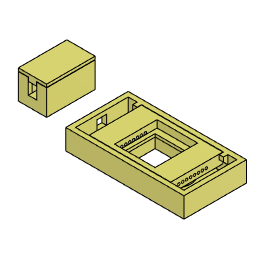
ESP07 Breadboard Adapter (Autodesk Fusion 360 design; units mm, degrees)
Autodesk Fusion 360 part; units mm, degrees
sketch "Footprint" plane through (0, 0, 0) normal (0, 0, 1) x (1, 0, 0)
  line L0 (21, 13.4625) -> (-21, 13.4625)
  line L1 (-21, 13.4625) -> (-21, -13.4625)
  line L2 (-21, -13.4625) -> (21, -13.4625)
  line L3 (21, -13.4625) -> (21, 13.4625)
  line L4 (21, 13.4625) -> (-21, -13.4625) construction
  line L5 (-21, 13.4625) -> (21, -13.4625) construction
  line L6 (10.45, 10.9625) -> (-10.45, 10.9625)
  line L7 (-10.45, 10.9625) -> (-10.45, -10.9625)
  line L8 (-10.45, -10.9625) -> (10.45, -10.9625)
  line L9 (10.45, -10.9625) -> (10.45, 10.9625)
  line L10 (10.45, 10.9625) -> (-10.45, -10.9625) construction
  line L11 (-10.45, 10.9625) -> (10.45, -10.9625) construction
  line L12 (-8.45, 7.9625) -> (8.45, 7.9625)
  line L13 (8.45, 7.9625) -> (8.45, -7.9625)
  line L14 (8.45, -7.9625) -> (-8.45, -7.9625)
  line L15 (-8.45, -7.9625) -> (-8.45, 7.9625)
  line L16 (-8.45, 7.9625) -> (8.45, -7.9625) construction
  line L17 (8.45, 7.9625) -> (-8.45, -7.9625) construction
  dimension "d16" = 21.925
  dimension "d17" = 20.9
  dimension "d18" = 2.5
  dimension "d19" = 10.55
  dimension "d20" = 3
  dimension "d21" = 2
  constraint perpendicular L0 L1
  constraint parallel L0 L2
  constraint parallel L1 L3
  constraint horizontal L0
  constraint coincident L4 origin
  constraint coincident L5 origin
  constraint perpendicular L6 L7
  constraint parallel L6 L8
  constraint parallel L7 L9
  constraint horizontal L6
  constraint coincident L10 origin
  constraint coincident L11 origin
  constraint perpendicular L12 L13
  constraint parallel L12 L14
  constraint parallel L13 L15
  constraint horizontal L12
  constraint coincident L16 origin
  constraint coincident L17 origin
  measures "d16" distance of L6.start L8.end
  measures "d17" distance of L7.end L8.end
  measures "d18" distance of L0 L6
  measures "d19" distance of L3 L9
  measures "d20" distance of L6 L12
  measures "d21" distance of L9 L13
extrude "Extrude1" add sketch "Footprint" against normal blind 1.5 contours L0 L1 L2 L3 | L6 L7 L8 L9 makes body 1
extrude "Extrude2" add sketch "Footprint" along normal blind 3.76 contours L0 L1 L2 L3 bodies 1
sketch "PogoPin Holes Profile" plane through (-10.45, 0, 0) normal (1, 0, 0) x (0, 1, 0)
  line L0 (-10.9625, 0) -> (10.9625, 0) construction
  line L1 (10.9625, 0) -> (10.9625, 3.76) construction
  line L2 (10.9625, 3.76) -> (-10.9625, 3.76) construction
  line L3 (-10.9625, 3.76) -> (-10.9625, 0) construction
  circle A0 centre (-9.2555, 0.8) radius 0.655
  circle A1 centre (-7.2355, 0.8) radius 0.655
  circle A2 centre (-5.2155, 0.8) radius 0.655
  circle A3 centre (-3.1955, 0.8) radius 0.655
  circle A4 centre (-1.1755, 0.8) radius 0.655
  circle A5 centre (0.8445, 0.8) radius 0.655
  circle A6 centre (2.8645, 0.8) radius 0.655
  circle A7 centre (4.8845, 0.8) radius 0.655
  dimension "d26" = 1.707
  dimension "d27" = 0.8
  dimension "d28" = 1.31
  dimension "d31" = 2.02
  dimension "d32" = 0
  measures "d26" distance of L3 A0.centre
  measures "d27" distance of L0 A0.centre
  measures "d28" diameter of A0
extrude "Extrude3" cut sketch "PogoPin Holes Profile" along normal through all and the other way through all bodies 1
sketch "Protector Sleve Profile" plane through (0, 0, -1.5) normal (0, 0, -1) x (1, 0, 0)
  line L0 (-28, 13.6175) -> (28, 13.6175)
  line L1 (28, 13.6175) -> (28, -13.6175)
  line L2 (28, -13.6175) -> (-28, -13.6175)
  line L3 (-28, -13.6175) -> (-28, 13.6175)
  line L4 (-28, 13.6175) -> (28, -13.6175) construction
  line L5 (28, 13.6175) -> (-28, -13.6175) construction
  line L6 (21, 13.4625) -> (-21, 13.4625)
  line L7 (30.5, -16.1175) -> (-30.5, -16.1175)
  line L8 (-30.5, -16.1175) -> (-30.5, 16.1175)
  line L9 (-30.5, 16.1175) -> (30.5, 16.1175)
  line L10 (30.5, 16.1175) -> (30.5, -16.1175)
  line L11 (21, -13.4625) -> (21, 13.4625)
  line L12 (-8.45, -7.9625) -> (-8.45, 7.9625)
  line L13 (8.45, 7.9625) -> (8.45, -7.9625)
  line L14 (8.45, -7.9625) -> (-8.45, -7.9625)
  line L15 (-8.45, 7.9625) -> (8.45, 7.9625)
  line L16 (-11.45, -9.1625) -> (11.45, -9.1625)
  line L17 (-11.45, 9.1625) -> (11.45, 9.1625)
  line L18 (0, -9.1625) -> (0, 9.1625) construction
  arc A0 (-11.45, 9.1625) -> (-11.45, -9.1625) centre (-7.9401, 0) ccw
  arc A1 (11.45, -9.1625) -> (11.45, 9.1625) centre (7.9401, 0) ccw
  point P0 (-21, 13.4625)
  point P1 (21, 13.4625)
  point P2 (21, -13.4625)
  point P3 (-21, -13.4625)
  point P4 (8.45, 7.9625)
  point P5 (-8.45, 7.9625)
  point P6 (-8.45, -7.9625)
  point P7 (8.45, -7.9625)
  dimension "d35" = 0.155
  dimension "d36" = 7
  dimension "d37" = -2.5
  dimension "d82" = 1.2
  dimension "d83" = 3
  constraint perpendicular L0 L1
  constraint parallel L0 L2
  constraint parallel L1 L3
  constraint horizontal L0
  constraint coincident L4 origin
  constraint coincident L5 origin
  constraint horizontal L16
  constraint horizontal L17
  constraint vertical L16.start L17.start
  constraint vertical L16.end L17.end
  constraint midpoint L16 L18.start
  constraint midpoint L17 L18.end
  constraint coincident origin L18
  constraint midpoint origin L18
  constraint equal A0 A1
  measures "d35" distance of L0 L6
  measures "d36" distance of P2 L1
  measures "d82" distance of L14 L16
  measures "d83" horizontal distance of P5 L17.start
extrude "Extrude4" add sketch "Protector Sleve Profile" against normal up to surface (5.26 mm away) separate body contours L7 L8 L9 L10 makes body 2
extrude "Extrude5" add sketch "Protector Sleve Profile" along normal blind 4 separate body makes body 3 at (-9.3333, -15.2842, -1.5) makes body 4 at (-11.5424, -0.2316, -1.5)
extrude "Extrude6" add sketch "Protector Sleve Profile" along normal blind 1.2 from surface at 4 contours L0 L1 L2 L3 | L7 L8 L9 L10 | L16 L17 A0 A1 bodies 1 3 2
combine "Combine1" operation add target body 3 tool bodies 2 4
sketch "Wires Cutout Profile" plane through (-28, 0, 0) normal (1, 0, 0) x (0, 1, 0)
  line L0 (-13.6175, 3.76) -> (-13.6175, -5.5) construction
  line L1 (-13.6175, -5.5) -> (13.6175, -5.5) construction
  line L2 (13.6175, -5.5) -> (13.6175, 3.76) construction
  line L3 (13.6175, 3.76) -> (-13.6175, 3.76) construction
  line L4 (-2.5, 1.63) -> (2.5, 1.63)
  line L5 (2.5, 1.63) -> (2.5, -3.37)
  line L6 (2.5, -3.37) -> (-2.5, -3.37)
  line L7 (-2.5, -3.37) -> (-2.5, 1.63)
  line L8 (13.6175, -0.87) -> (2.5, -0.87) construction
  line L9 (-2.5, -0.87) -> (-13.6175, -0.87) construction
  dimension "d46" = 5
  dimension "d47" = 5
  constraint horizontal L4
  constraint vertical L5
  constraint horizontal L6
  constraint vertical L7
  constraint midpoint L2 L8.start
  constraint midpoint L5 L8.end
  constraint midpoint L7 L9.start
  constraint midpoint L0 L9.end
  constraint equal L8 L9
  constraint collinear L8 L9
  measures "d46" distance of L5.end L6.end
  measures "d47" distance of L4.end L5.end
extrude "Extrude7" cut sketch "Wires Cutout Profile" against normal through all bodies 3
sketch "Connector Profile" plane through (0, 0, 0) normal (0, 0, 1) x (1, 0, 0)
  line L0 (-59.4813, 13.4549) -> (-44.8813, 13.4549)
  line L1 (-44.8813, 13.4549) -> (-44.8813, -11.5851)
  line L2 (-44.8813, -11.5851) -> (-59.4813, -11.5851)
  line L3 (-59.4813, -11.5851) -> (-59.4813, 13.4549)
  line L4 (-57.4813, 11.4549) -> (-54.3813, 11.4549)
  line L5 (-54.3813, 11.4549) -> (-54.3813, -9.5851)
  line L6 (-54.3813, -9.5851) -> (-57.4813, -9.5851)
  line L7 (-57.4813, -9.5851) -> (-57.4813, 11.4549)
  line L8 (-49.9813, 11.4549) -> (-46.8813, 11.4549)
  line L9 (-46.8813, 11.4549) -> (-46.8813, -9.5851)
  line L10 (-46.8813, -9.5851) -> (-49.9813, -9.5851)
  line L11 (-49.9813, -9.5851) -> (-49.9813, 11.4549)
  line L12 (-49.9813, -9.5851) -> (-54.3813, -9.5851)
  line L13 (-49.9813, 11.4549) -> (-54.3813, 11.4549)
  line L14 (-49.9813, -9.5851) -> (-49.9813, -11.5851)
  line L15 (-54.3813, -9.5851) -> (-54.3813, -11.5851)
  circle A0 centre (-55.9313, 9.6849) radius 0.7
  line L16 (-55.9313, 9.6849) -> (-55.9313, 11.4549) construction
  circle A1 centre (-55.9313, 7.1849) radius 0.7
  circle A2 centre (-55.9313, 4.6849) radius 0.7
  circle A3 centre (-55.9313, 2.1849) radius 0.7
  circle A4 centre (-55.9313, -0.3151) radius 0.7
  circle A5 centre (-55.9313, -2.8151) radius 0.7
  circle A6 centre (-55.9313, -5.3151) radius 0.7
  circle A7 centre (-55.9313, -7.8151) radius 0.7
  circle A8 centre (-48.4313, 9.6849) radius 0.7
  line L17 (-48.4313, 9.6849) -> (-48.4313, 11.4549) construction
  circle A9 centre (-48.4313, 7.1849) radius 0.7
  circle A10 centre (-48.4313, 4.6849) radius 0.7
  circle A11 centre (-48.4313, 2.1849) radius 0.7
  circle A12 centre (-48.4313, -0.3151) radius 0.7
  circle A13 centre (-48.4313, -2.8151) radius 0.7
  circle A14 centre (-48.4313, -5.3151) radius 0.7
  circle A15 centre (-48.4313, -7.8151) radius 0.7
  dimension "d49" = 3.1
  dimension "d51" = 2
  dimension "d52" = 2
  dimension "d54" = 2
  dimension "d55" = 2
  dimension "d63" = 1.4
  dimension "d64" = 1.77
  dimension "d67" = 0
  dimension "d68" = -2.5
  dimension "d69" = 1.77
  dimension "d70" = 7.5
  constraint horizontal L0
  constraint vertical L1
  constraint horizontal L2
  constraint vertical L3
  constraint horizontal L4
  constraint vertical L5
  constraint horizontal L6
  constraint vertical L7
  constraint horizontal L8
  constraint vertical L9
  constraint horizontal L10
  constraint vertical L11
  constraint equal L4 L8
  constraint equal L5 L9
  constraint collinear L4 L8
  constraint coincident L2 L14.end
  constraint perpendicular L2 L14
  constraint coincident L2 L15.end
  constraint perpendicular L2 L15
  constraint coincident A0.centre L16.start
  constraint midpoint L4 L16.end
  constraint perpendicular L4 L16
  constraint equal A0 A8
  constraint coincident A8.centre L17.start
  constraint midpoint L8 L17.end
  constraint perpendicular L8 L17
  constraint equal L16 L17
  measures "d49" distance of L4.start L4.end
  measures "d51" distance of L1 L9
  measures "d52" distance of L3 L7
  measures "d54" distance of L0 L8
  measures "d55" distance of L2 L10
  measures "d63" diameter of A0
  measures "d64" distance of L4 A0.centre
  measures "d69" distance of L6 A7.centre
  measures "d70" distance of A0.centre A8.centre
extrude "Extrude8" add sketch "Connector Profile" against normal blind 1.2 separate body makes body 5
extrude "Extrude9" add sketch "Connector Profile" along normal blind 4 contours L0 L1 L2 L3 L4 L6 L7 L8 L9 L10 L13 L14 L15 | L2 L12 L14 L15 | L5 L11 L12 L13 bodies 5
extrude "Breadboard Connector" add sketch "Connector Profile" along normal blind 8 from surface at 4 contours L0 L1 L2 L3 L4 L6 L7 L8 L9 L10 L13 L14 L15 bodies 5
sketch "Lid Profile" plane through (0, 0, 0) normal (0, 0, 1) x (1, 0, 0)
  line L0 (-57.4813, 11.4549) -> (-46.8813, 11.4549) construction
  line L1 (-46.8813, 11.4549) -> (-46.8813, -9.5851) construction
  line L2 (-46.8813, -9.5851) -> (-57.4813, -9.5851) construction
  line L3 (-57.4813, -9.5851) -> (-57.4813, 11.4549) construction
  line L4 (-59.4813, 13.4549) -> (-44.8813, 13.4549)
  line L5 (-44.8813, 13.4549) -> (-44.8813, -11.5851)
  line L6 (-44.8813, -11.5851) -> (-59.4813, -11.5851)
  line L7 (-59.4813, -11.5851) -> (-59.4813, 13.4549)
  line L8 (-57.1484, -9.4301) -> (-57.1484, 11.2999)
  line L9 (-57.1484, 11.2999) -> (-47.0363, 11.2999)
  line L10 (-47.0363, 11.2999) -> (-47.0363, -9.4301)
  line L11 (-50.1363, -11.5851) -> (-50.1363, -9.4301)
  line L12 (-54.2263, -11.5851) -> (-54.2263, -9.4301)
  line L13 (-47.0363, -9.4301) -> (-50.1363, -9.4301)
  line L14 (-54.2263, -9.4301) -> (-57.1484, -9.4301)
  point P0 (-59.4813, 13.4549)
  point P1 (-44.8813, 13.4549)
  point P2 (-57.4813, 11.4549)
  point P3 (-57.4813, -9.5851)
  point P4 (-46.8813, -9.5851)
  point P5 (-46.8813, 11.4549)
  point P6 (-59.4813, -11.5851)
  point P7 (-44.8813, -11.5851)
  point P8 (-49.9813, -11.5851)
  point P9 (-54.3813, -11.5851)
  dimension "d78" = 0.155
  dimension "d79" = 0.155
  constraint horizontal L0
  constraint vertical L1
  constraint horizontal L2
  constraint vertical L3
  constraint coincident P4 L1.end
  constraint coincident P2 L0.start
  constraint horizontal L4
  constraint vertical L5
  constraint horizontal L6
  constraint vertical L7
  constraint coincident P7 L5.end
  constraint coincident P0 L4.start
  constraint coincident L6 L11.start
  constraint perpendicular L11 L13
  constraint coincident L6 L12.start
  constraint coincident L12.end L13
  constraint perpendicular L12 L13
  constraint parallel L3 L8
  constraint parallel L0 L9
  constraint parallel L1 L10
  constraint parallel L2 L13
  constraint collinear L13 L14
  measures "d78" distance of P9 L12
  measures "d79" distance of P8 L11
extrude "Extrude11" add sketch "Lid Profile" against normal blind 2 from surface at 12.155 separate body contours L6 L8 L9 L10 L11 L12 L13 L14 makes body 6
extrude "Extrude12" add sketch "Lid Profile" along normal blind 1.5 from surface at 12.155 bodies 6
sketch "Guide Profile" plane through (0, 13.6175, 0) normal (0, -1, 0) x (1, 0, 0)
  line L0 (-21, -1.5) -> (-21, 3.76)
  line L1 (21, -1.5) -> (21, 3.76)
  line L2 (-23.415, 3.76) -> (-21.155, 3.76)
  line L3 (-21.155, 3.76) -> (-21.155, 1.5)
  line L4 (-21.155, 1.5) -> (-23.415, 1.5)
  line L5 (-23.415, 1.5) -> (-23.415, 3.76)
  line L6 (21.155, 3.76) -> (23.415, 3.76)
  line L7 (23.415, 3.76) -> (23.415, 1.5)
  line L8 (23.415, 1.5) -> (21.155, 1.5)
  line L9 (21.155, 1.5) -> (21.155, 3.76)
  dimension "d84" = 0.155
  dimension "d85" = 0.155
  dimension "d86" = 2.26
  dimension "d87" = 2.26
  constraint horizontal L2
  constraint vertical L3
  constraint horizontal L4
  constraint vertical L5
  constraint horizontal L6
  constraint vertical L7
  constraint horizontal L8
  constraint vertical L9
  constraint equal L2 L6
  constraint equal L5 L7
  constraint horizontal L0.end L2.end
  constraint horizontal L1.end L6.start
  measures "d84" distance of L0 L3
  measures "d85" distance of L1 L9
  measures "d86" distance of L2.start L4.end
  measures "d87" distance of L2.start L2.end
extrude "Extrude13" add sketch "Guide Profile" along normal blind 2.26 bodies 3
chamfer "Chamfer1" distance 2.26 angle 45 2 edges at (-22.285, 13.6175, 1.5) (22.285, 13.6175, 1.5) on bodies 3
equation "ESP_Width = 16.06 mm" comment "The width is across the side that has the antena"
equation "ESP_Height = 21.5 mm" comment "The height is across the side that has the castellated pins"
equation "ESP_Thikness = 3.42 mm" comment "The thikness of the hole device (including the PCB and the metal radio case"
equation "ESP_PCBOnlyThikness = 1.06 mm" comment "The thikness PCB on which all the components are soldered"
equation "ESP_CastelatedPadWidth = 1 mm" comment "The width of the pad (measured along the side of the device)"
equation "ESP_CastelatedPadDepth = 1.6 mm" comment "The distance each pad extends inward"
equation "ESP_CastelatedPadHoleDiameter = 0.6 mm" comment "The diameter of the hole in the pad (same as the diameter of the cutout that makes it 'castelated'"
equation "ESP_CastelatedPadSpacing = 1.02 mm" comment "The distance between two consecutive pads"
equation "ESP_CastelatedPadBottomSpacing = 5.2 mm" comment "The distance between the last pad and the edge (where the antena is)"
equation "Tolerance = 0.17 mm"
equation "Tolerance_Tight = 0.155 mm"
equation "Tolerance_PressFitLight = 0.12 mm"
equation "PogoPin_Length = 16.05 mm" comment "The total length of a pogo pin"
equation "PogoPin_Diameter = 1 mm" comment "The diameter of the pogo pin (at its thickest)"
equation "PogoPin_RetractableLength = 3 mm" comment "The length of the pin that can be pushed in"
equation "d16 = ESP_Height + 2.5 * Tolerance"
equation "d17 = ESP_Width + 1.5 * PogoPin_RetractableLength + 2 * Tolerance"
equation "d19 = PogoPin_Length - PogoPin_RetractableLength - 2.5 mm"
equation "d22 = -1.5 mm"
equation "d24 = ESP_Thikness + 2 * Tolerance"
equation "d26 = ( ESP_CastelatedPadSpacing / 2 + 1.1 * Tolerance ) + ( ESP_CastelatedPadWidth + ESP_CastelatedPadSpacing ) / 2"
equation "d27 = PogoPin_Diameter / 2 + 0.3 mm"
equation "d28 = PogoPin_Diameter + 2 * Tolerance_Tight"
equation "d31 = ESP_CastelatedPadWidth + ESP_CastelatedPadSpacing"
equation "d35 = Tolerance_Tight"
equation "d51 = d52"
equation "d54 = d51"
equation "d55 = d54"
equation "d69 = d64"
equation "d72 = Tolerance_Tight"
equation "d78 = Tolerance_Tight"
equation "d79 = Tolerance_Tight"
equation "d84 = Tolerance_Tight"
equation "d85 = d84"
equation "d86 = d22 + d24"
equation "d87 = d86"
equation "d88 = d22 + d24"
equation "d90 = d22 + d24"
named bodies: "Pins Body", "Protector Sleve Body", "Protector Sleve", "Connector", "Connector Lid"
